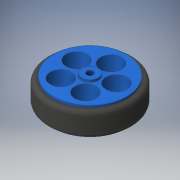
# Autodesk Inventor part: Rueda
Saved by Autodesk Inventor 2016 SP2 (Build 200236200, 236)
## iProperties
Created: 2017-06-02
Part Number: Rueda
Material: Caucho, butilo(1)
Document SubType Name: Modeling
Designer: ssant
Density: 0.12 g/cm^3
Appearance: Goma - Negro(1)
Author: ssant
Autodesk Inventor part; units mm, degrees
ref_plane "YZ Plane" through (0, 0, 0) normal (1, 0, 0) x (0, 1, 0)
ref_plane "XY Plane" through (0, 0, 0) normal (0, 0, 1) x (1, 0, 0)
sketch "Boceto1" plane through (0, 0, 0) normal (0, 1, 0) x (-1, 0, 0)
  circle A0 centre (0, 0) radius 17.5
  dimension "d0" = 35
  constraints: 1 centre point, 1 coincident
  measures "d0" diameter of A0
extrude "Extrusión1" add sketch "Boceto1" along normal blind 13
sketch "Boceto2" plane through (0, 13, 0) normal (0, 1, 0) x (1, 0, 0)
  circle A0 centre (0, 0) radius 17.5 projected
  circle A1 centre (0, 0) radius 4
  circle A2 centre (0, 10) radius 5
  circle A3 centre (-9.5106, 3.0902) radius 5
  circle A4 centre (-5.8779, -8.0902) radius 5
  circle A5 centre (5.8779, -8.0902) radius 5
  circle A6 centre (9.5106, 3.0902) radius 5
  circle A7 centre (0, 0) radius 17.5 projected
  dimension "d3" = 8
  dimension "d4" = 10
  dimension "d5" = 10
  dimension "d8" = 360
  constraints: 6 centre point, 1 coincident, 1 concentric, 1 vertical alignment, 11 other
  measures "d3" diameter of A1
  measures "d4" diameter of A2
  measures "d5" distance of A2.centre point (0, 0)
extrude "Extrusión2" add sketch "Boceto2" along normal blind 1 contours A1
extrude "Extrusión3" cut sketch "Boceto2" against normal blind 15 contours A2 | A3 | A4 | A5 | A6
sketch "Boceto3" plane through (0, 14, 0) normal (0, 1, 0) x (1, 0, 0)
  circle A0 centre (0, 0) radius 1.5
  dimension "d14" = 3
  constraints: 1 centre point, 1 coincident
  measures "d14" diameter of A0
extrude "Extrusión4" cut sketch "Boceto3" against normal blind 15
ref_plane "Plano de trabajo1" through (0, 1, 0) normal (0, 1, 0) x (-1, 0, 0)
sketch "Boceto4" plane through (0, 1, 0) normal (0, 1, 0) x (-1, 0, 0)
  circle A0 centre (5.8779, 8.0902) radius 5 projected
  circle A1 centre (-9.5106, -3.0902) radius 5 projected
  circle A2 centre (9.5106, -3.0902) radius 5 projected
  circle A3 centre (0, -10) radius 5 projected
  circle A4 centre (-5.8779, 8.0902) radius 5 projected
  circle A5 centre (0, 0) radius 4 projected
  circle A6 centre (0, 0) radius 17.5 projected
  circle A7 centre (0, 0) radius 20
  dimension "d18" = 40
  constraints: 1 centre point, 1 coincident
  measures "d18" diameter of A7
extrude "Extrusión5" add sketch "Boceto4" along normal blind 11 contours A7
fillet "Empalme1" radius 2 2 edges at (20, 12, 0) (20, 1, 0)
